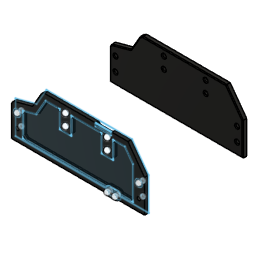
PSU Mounting plates (Autodesk Fusion 360 design; units mm, degrees)
Autodesk Fusion 360 part; units mm, degrees
sketch "sketch 1169" plane through (0, 0, 781.75) normal (0, 0, 1) x (1, 0, 0)
  circle A0 centre (305.3, -33.602) radius 2.25
  circle A1 centre (305.3, -51.602) radius 2.25
  circle A2 centre (145.3, -33.602) radius 2.25
  circle A3 centre (145.3, -51.602) radius 2.25
  line L0 (137.8, -66.602) -> (312.8, -66.602)
  line L1 (137.8, -66.602) -> (312.8, -66.602)
  line L2 (312.8, -66.602) -> (312.8, -23.602)
  line L3 (312.8, -23.602) -> (291, 6.398)
  line L4 (178.5, 6.398) -> (291, 6.398)
  line L5 (165.4582, -16.191) -> (178.5, 6.398)
  line L6 (137.8, -23.602) -> (165.4582, -16.191)
  line L7 (137.8, -66.602) -> (137.8, -23.602)
extrude "Extrude1" add sketch "sketch 1169" along normal blind 5.25 makes body 1
sketch "sketch 1213" plane through (0, 0, 787) normal (0, 0, 1) x (1, 0, 0)
  circle A0 centre (264, -1.877) radius 2.25
  circle A1 centre (264, -1.877) radius 2.25
  circle A2 centre (209, -16.877) radius 2.25
  circle A3 centre (209, -16.877) radius 2.25
  circle A4 centre (209, -1.877) radius 2.25
  circle A5 centre (209, -1.877) radius 2.25
  circle A6 centre (264, -16.877) radius 2.25
  circle A7 centre (264, -16.877) radius 2.25
extrude "Extrude3" cut sketch "sketch 1213" against normal blind 5.25 bodies 1
chamfer "Chamfer2" distance 1.75 angle 45 4 edges at (206.9023, -1.0634, 787) (206.9023, -16.0634, 787) (261.9023, -1.0634, 787) (261.9023, -16.0634, 787) on bodies 1
sketch "sketch 1249" plane through (0, 0, 787) normal (0, 0, 1) x (1, 0, 0)
  line L0 (170.4001, -22.6314) -> (152.8, -27.3474)
  line L1 (152.8, -27.3474) -> (152.8, -59.102)
  line L2 (152.8, -59.102) -> (297.8, -59.102)
  line L3 (297.8, -59.102) -> (297.8, -15.7182)
  line L4 (287.1789, -1.102) -> (297.8, -15.7182)
  line L5 (271.5, -1.102) -> (287.1789, -1.102)
  line L6 (271.5, -24.377) -> (271.5, -1.102)
  line L7 (256.5, -24.377) -> (271.5, -24.377)
  line L8 (256.5, -1.102) -> (256.5, -24.377)
  line L9 (216.5, -1.102) -> (256.5, -1.102)
  line L10 (216.5, -24.377) -> (216.5, -1.102)
  line L11 (201.5, -24.377) -> (216.5, -24.377)
  line L12 (201.5, -1.102) -> (201.5, -24.377)
  line L13 (182.8301, -1.102) -> (201.5, -1.102)
  line L14 (170.4001, -22.6314) -> (182.8301, -1.102)
extrude "Extrude2" cut sketch "sketch 1249" against normal blind 3.75 bodies 1
chamfer "Chamfer1" distance 3.5 angle 45 11 edges at (152.8, -27.3474, 785.125) (152.8, -59.102, 785.125) (297.8, -59.102, 785.125) (201.5, -1.102, 785.125) (201.5, -24.377, 785.125) (216.5, -24.377, 785.125) (216.5, -1.102, 785.125) (256.5, -1.102, 785.125) (256.5, -24.377, 785.125) (271.5, -24.377, 785.125) (271.5, -1.102, 785.125) on bodies 1
chamfer "Chamfer3" distance 1 angle 45 1 faces at (221.2, -47.527, 783.25) on bodies 1
chamfer "Chamfer4" distance 2.5 angle 45 2 edges at (137.8, -23.602, 784.375) (178.5, 6.398, 784.375) on bodies 1
chamfer "Chamfer5" distance 1 angle 45 1 faces at (219.9286, -50.7745, 781.75) on bodies 1
mirror "Mirror1" about plane through (219.5, -44.102, 719.75) normal (0, 0, 1) of bodies 1 makes body 2
sketch "sketch 1303" plane through (0, 0, 787) normal (0, 0, 1) x (1, 0, 0)
  line L0 (268.8583, 2.548) -> (248.55, 2.548)
  line L1 (268.8583, 6.398) -> (268.8583, 2.548)
  line L2 (248.55, 6.398) -> (268.8583, 6.398)
  line L3 (248.55, 6.398) -> (268.8583, 6.398)
  line L4 (248.55, 2.548) -> (248.55, 6.398)
extrude "Extrude4" cut sketch "sketch 1303" against normal blind 6 bodies 1
chamfer "Chamfer6" distance 1 angle 45 4 edges at (248.55, 2.548, 784.375) (268.8583, 2.548, 784.375) (268.8583, 6.398, 784.875) (248.55, 6.398, 784.875) on bodies 1
sketch "sketch 1325" plane through (0, 0, 787) normal (0, 0, 1) x (1, 0, 0)
  circle A0 centre (145.3, -33.602) radius 4.125
  circle A1 centre (305.3, -33.602) radius 4.125
extrude "Extrude5" cut sketch "sketch 1325" against normal blind 1.25 bodies 1
chamfer "Chamfer7" distance 1.875 angle 45 2 edges at (147.3977, -32.7884, 785.75) (307.3977, -32.7884, 785.75) on bodies 1
sketch "sketch 1342" plane through (0, 0, 787) normal (0, 0, 1) x (1, 0, 0)
  arc A0 (267, -56.852) -> (267, -66.352) centre (267, -61.602) ccw
  line L0 (267, -66.352) -> (277, -66.352)
  arc A1 (277, -66.352) -> (277, -56.852) centre (277, -61.602) ccw
  line L1 (267, -56.852) -> (277, -56.852)
extrude "Extrude6" add sketch "sketch 1342" along normal blind -4 and the other way blind -3 bodies 1
chamfer "Chamfer8" distance 1 angle 45 3 edges at (265.277, -57.1756, 783.25) (272, -56.852, 783.25) (278.723, -57.1756, 783.25) on bodies 1
sketch "sketch 1367" plane through (0, 0, 790) normal (0, 0, 1) x (1, 0, 0)
  circle A0 centre (267, -61.602) radius 1.875
  circle A1 centre (277, -61.602) radius 1.875
extrude "Extrude7" cut sketch "sketch 1367" against normal blind 8.25 bodies 1
chamfer "Chamfer9" distance 0.5 angle 45 4 edges at (272, -56.852, 790) (262.25, -61.602, 790) (272, -66.352, 790) (281.75, -61.602, 790) on bodies 1
equation "d2913 = -5.25 mm + 1.5 mm"
